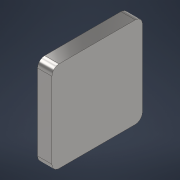
# Autodesk Inventor part: Retranslator
Saved by Autodesk Inventor 2022 (Build 260153000, 153)
## iProperties
Created: 2022-07-14
Part Number: Retranslator
Material: Iron, Malleable
Document SubType Name: Modeling
Designer: ForseFire
Density: 7.15 g/cm^3
Appearance: Semi-Polished
Author: ForseFire
Autodesk Inventor part; units mm, degrees
ref_plane "YZ Plane" through (0, 0, 0) normal (1, 0, 0) x (0, 1, 0)
ref_plane "XZ Plane" through (0, 0, 0) normal (0, 1, 0) x (-1, 0, 0)
ref_plane "XY Plane" through (0, 0, 0) normal (0, 0, 1) x (1, 0, 0)
sketch "Sketch1" plane through (0, 0, 0) normal (1, 0, 0) x (0, 1, 0)
  line L0 (-12.6, -12.6) -> (12.6, -12.6)
  line L1 (12.6, -12.6) -> (12.6, 12.6)
  line L2 (12.6, 12.6) -> (-12.6, 12.6)
  line L3 (-12.6, 12.6) -> (-12.6, -12.6)
  line L4 (-12.6, -12.6) -> (12.6, 12.6) construction
  line L5 (12.6, -12.6) -> (-12.6, 12.6) construction
  point P0 (0, 0)
  dimension "d0" = 25.2
  dimension "d1" = 25.2
  constraints: 12 end point, 2 midpoint, 2 parallel, 1 horizontal, 1 perpendicular
  measures "d0" distance of L2.end L1.end
  measures "d1" distance of L0.end L1.end
extrude "Extrusion1" add sketch "Sketch1" along normal blind 4
fillet "Fillet1" radius 2 4 edges at (2, 12.6, 12.6) (2, 12.6, -12.6) (2, -12.6, -12.6) (2, -12.6, 12.6)
body "Solid1"
